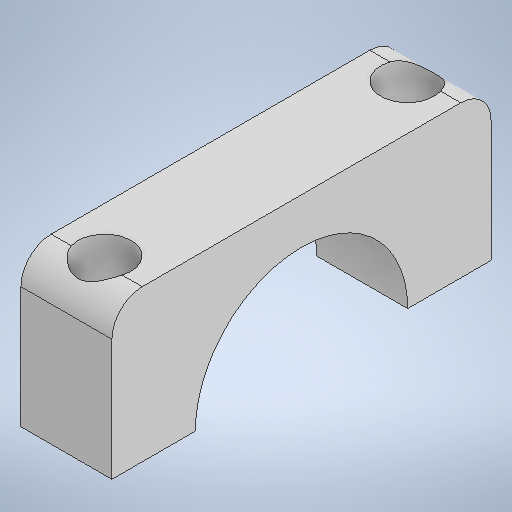
# Autodesk Inventor part: Base
Saved by Autodesk Inventor 2025 (Build 290162000, 162)
## iProperties
Created: 2024-06-05
Part Number: Base
Material: Générique
Document SubType Name: Modeling
Designer: luc4s
Density: 1 g/cm^3
Appearance: Par défaut
Author: luc4s
Autodesk Inventor part; units mm, degrees
ref_plane "YZ Plane" through (0, 0, 0) normal (1, 0, 0) x (0, 1, 0)
ref_plane "XZ Plane" through (0, 0, 0) normal (0, 1, 0) x (-1, 0, 0)
ref_plane "XY Plane" through (0, 0, 0) normal (0, 0, 1) x (1, 0, 0)
sketch "Esquisse1" plane through (0, 0, 0) normal (1, 0, 0) x (0, 1, 0)
  arc A0 (0, -7) -> (0, 7) centre (0, 0) ccw
  line L0 (0, 6.2947) -> (0, -6.5718) construction
  line L1 (0, 7) -> (0, 12.5)
  line L2 (0, 12.5) -> (10, 12.5)
  line L3 (10, -12.5) -> (0, -12.5)
  line L4 (0, -12.5) -> (0, -7)
  line L5 (10, 12.5) -> (10, -12.5)
  dimension "d16" = 7
  dimension "d17" = 25
  dimension "d31" = 10
  constraints: 12 end point, 5 point on line, 2 equal length, 2 point on circle, 2 vertical, 1 centre point, 1 coincident, 1 collinear, 1 perpendicular
  measures "d16" radius of A0
  measures "d17" distance of L3.end L1.end
  measures "d31" distance of L3.start L3.end
extrude "Extrusion1" add sketch "Esquisse1" along normal blind 6
sketch "Esquisse2" plane through (0, 0, -12.5) normal (0, -1, 0) x (1, 0, 0)
  circle A0 centre (3, 2.5187) radius 1.75
  line L0 (0, -7) -> (0, 2) projected
  line L1 (6, -4) -> (6, 22) projected
  line L2 (6, 0.0034) -> (0, 5.034) construction
  line L3 (0, -4) -> (0, 22) projected
  line L4 (0, 0.0034) -> (6, 5.034) construction
  point P0 (0, 12.5)
  point P1 (0, -5)
  dimension "d28" = 3.5
  constraints: 4 end point, 4 point on line, 2 midpoint, 1 centre point
  measures "d28" diameter of A0
extrude "Extrusion2" cut sketch "Esquisse2" against normal blind 15
mirror "Mise en miroir1" about plane through (0, 0, 0) normal (0, 0, 1) of "Extrusion2"
fillet "Congé4" radius 2 2 edges at (3, 10, -12.5) (3, 10, 12.5)
